Autodesk Fusion 360 part; units mm, degrees
(part 2 of 2)
sketch "Sketch5 (5)" plane through (85, 0, 0) normal (1, 0, 0) x (0, 0, -1) in component "Top"
  line L0 (-100, 190) -> (-100, 195)
  line L1 (-100, 195) -> (-145, 195)
  line L2 (-145, 195) -> (-145, 156)
  line L3 (-145, 156) -> (-150, 156)
  line L4 (-150, 156) -> (-150, 117)
  line L5 (-150, 117) -> (-145, 117)
  line L6 (-145, 117) -> (-145, 78)
  line L7 (-145, 78) -> (-150, 78)
  line L8 (-150, 78) -> (-150, 39)
  line L9 (-150, 39) -> (-145, 39)
  line L10 (-145, 39) -> (-145, 5)
  line L11 (-145, 5) -> (-100, 5)
  line L12 (-100, 5) -> (-100, 0)
  line L13 (-100, 0) -> (-50, 0)
  line L14 (-50, 0) -> (-50, 5)
  line L15 (-50, 5) -> (-5, 5)
  line L16 (-5, 5) -> (-5, 39)
  line L17 (-5, 39) -> (0, 39)
  line L18 (0, 39) -> (0, 78)
  line L19 (0, 78) -> (-5, 78)
  line L20 (-5, 78) -> (-5, 117)
  line L21 (-5, 117) -> (0, 117)
  line L22 (0, 117) -> (0, 156)
  line L23 (0, 156) -> (-5, 156)
  line L24 (-5, 156) -> (-5, 195)
  line L25 (-5, 195) -> (-50, 195)
  line L26 (-50, 195) -> (-50, 190)
  line L27 (-50, 190) -> (-100, 190)
  line L28 (-85, 117) -> (-80, 117)
  line L29 (-80, 117) -> (-80, 78)
  line L30 (-80, 78) -> (-85, 78)
  line L31 (-85, 78) -> (-85, 117)
sketch "Sketch6 (3)" plane through (85, 0, 0) normal (1, 0, 0) x (0, 0, -1) in component "Top"
  line L0 (-100, 190) -> (-100, 195)
  line L1 (-100, 195) -> (-145, 195)
  line L2 (-145, 195) -> (-145, 156)
  line L3 (-145, 156) -> (-150, 156)
  line L4 (-150, 156) -> (-150, 117)
  line L5 (-150, 117) -> (-145, 117)
  line L6 (-145, 117) -> (-145, 78)
  line L7 (-145, 78) -> (-150, 78)
  line L8 (-150, 78) -> (-150, 39)
  line L9 (-150, 39) -> (-145, 39)
  line L10 (-145, 39) -> (-145, 5)
  line L11 (-145, 5) -> (-100, 5)
  line L12 (-100, 5) -> (-100, 0)
  line L13 (-100, 0) -> (-50, 0)
  line L14 (-50, 0) -> (-50, 5)
  line L15 (-50, 5) -> (-5, 5)
  line L16 (-5, 5) -> (-5, 39)
  line L17 (-5, 39) -> (0, 39)
  line L18 (0, 39) -> (0, 78)
  line L19 (0, 78) -> (-5, 78)
  line L20 (-5, 78) -> (-5, 117)
  line L21 (-5, 117) -> (0, 117)
  line L22 (0, 117) -> (0, 156)
  line L23 (0, 156) -> (-5, 156)
  line L24 (-5, 156) -> (-5, 195)
  line L25 (-5, 195) -> (-50, 195)
  line L26 (-50, 195) -> (-50, 190)
  line L27 (-50, 190) -> (-100, 190)
  line L28 (-85, 117) -> (-80, 117)
  line L29 (-80, 117) -> (-80, 78)
  line L30 (-80, 78) -> (-85, 78)
  line L31 (-85, 78) -> (-85, 117)
sketch "Sketch7 (3)" plane through (85, 0, 0) normal (1, 0, 0) x (0, 0, -1) in component "Top"
  line L0 (-100, 190) -> (-100, 195)
  line L1 (-100, 195) -> (-145, 195)
  line L2 (-145, 195) -> (-145, 156)
  line L3 (-145, 156) -> (-150, 156)
  line L4 (-150, 156) -> (-150, 117)
  line L5 (-150, 117) -> (-145, 117)
  line L6 (-145, 117) -> (-145, 78)
  line L7 (-145, 78) -> (-150, 78)
  line L8 (-150, 78) -> (-150, 39)
  line L9 (-150, 39) -> (-145, 39)
  line L10 (-145, 39) -> (-145, 5)
  line L11 (-145, 5) -> (-100, 5)
  line L12 (-100, 5) -> (-100, 0)
  line L13 (-100, 0) -> (-50, 0)
  line L14 (-50, 0) -> (-50, 5)
  line L15 (-50, 5) -> (-5, 5)
  line L16 (-5, 5) -> (-5, 39)
  line L17 (-5, 39) -> (0, 39)
  line L18 (0, 39) -> (0, 78)
  line L19 (0, 78) -> (-5, 78)
  line L20 (-5, 78) -> (-5, 117)
  line L21 (-5, 117) -> (0, 117)
  line L22 (0, 117) -> (0, 156)
  line L23 (0, 156) -> (-5, 156)
  line L24 (-5, 156) -> (-5, 195)
  line L25 (-5, 195) -> (-50, 195)
  line L26 (-50, 195) -> (-50, 190)
  line L27 (-50, 190) -> (-100, 190)
  line L28 (-85, 117) -> (-80, 117)
  line L29 (-80, 117) -> (-80, 78)
  line L30 (-80, 78) -> (-85, 78)
  line L31 (-85, 78) -> (-85, 117)
sketch "Div2" plane through (85, 0, 0) normal (1, 0, 0) x (0, 0, -1)
  line L0 (-100, 190) -> (-100, 195)
  line L1 (-100, 195) -> (-145, 195)
  line L2 (-145, 195) -> (-145, 156)
  line L3 (-145, 156) -> (-150, 156)
  line L4 (-150, 156) -> (-150, 117)
  line L5 (-150, 117) -> (-145, 117)
  line L6 (-145, 117) -> (-145, 78)
  line L7 (-145, 78) -> (-150, 78)
  line L8 (-150, 78) -> (-150, 39)
  line L9 (-150, 39) -> (-145, 39)
  line L10 (-145, 39) -> (-145, 5)
  line L11 (-145, 5) -> (-100, 5)
  line L12 (-100, 5) -> (-100, 0)
  line L13 (-100, 0) -> (-50, 0)
  line L14 (-50, 0) -> (-50, 5)
  line L15 (-50, 5) -> (-5, 5)
  line L16 (-5, 5) -> (-5, 39)
  line L17 (-5, 39) -> (0, 39)
  line L18 (0, 39) -> (0, 78)
  line L19 (0, 78) -> (-5, 78)
  line L20 (-5, 78) -> (-5, 117)
  line L21 (-5, 117) -> (0, 117)
  line L22 (0, 117) -> (0, 156)
  line L23 (0, 156) -> (-5, 156)
  line L24 (-5, 156) -> (-5, 195)
  line L25 (-5, 195) -> (-50, 195)
  line L26 (-50, 195) -> (-50, 190)
  line L27 (-50, 190) -> (-100, 190)
  line L28 (-85, 117) -> (-80, 117)
  line L29 (-80, 117) -> (-80, 78)
  line L30 (-80, 78) -> (-85, 78)
  line L31 (-85, 78) -> (-85, 117)
sketch "Div4" plane through (255, 0, 85) normal (0, 0, 1) x (1, 0, 0)
  line L0 (-250, 5) -> (-237.5, 5)
  line L1 (-237.5, 5) -> (-237.5, 0)
  line L2 (-237.5, 0) -> (-187.5, 0)
  line L3 (-187.5, 0) -> (-187.5, 5)
  line L4 (-187.5, 5) -> (-175, 5)
  line L5 (-175, 5) -> (-175, 78)
  line L6 (-175, 78) -> (-170, 78)
  line L7 (-170, 78) -> (-170, 117)
  line L8 (-170, 117) -> (-175, 117)
  line L9 (-175, 117) -> (-175, 190)
  line L10 (-175, 190) -> (-250, 190)
  line L11 (-250, 190) -> (-250, 117)
  line L12 (-250, 117) -> (-255, 117)
  line L13 (-255, 117) -> (-255, 78)
  line L14 (-255, 78) -> (-250, 78)
  line L15 (-250, 78) -> (-250, 5)
sketch "Bottom" plane through (0, 0, 0) normal (0, -1, 0) x (1, 0, 0)
  line L0 (67.5, 85) -> (67.5, 80)
  line L1 (67.5, 80) -> (17.5, 80)
  line L2 (17.5, 80) -> (17.5, 85)
  line L3 (17.5, 85) -> (67.5, 85)
  line L4 (80, 50) -> (80, 100)
  line L5 (80, 100) -> (85, 100)
  line L6 (85, 100) -> (85, 50)
  line L7 (85, 50) -> (80, 50)
  line L8 (295, 50) -> (295, 100)
  line L9 (295, 100) -> (300, 100)
  line L10 (300, 100) -> (300, 145)
  line L11 (300, 145) -> (250, 145)
  line L12 (250, 145) -> (250, 150)
  line L13 (250, 150) -> (200, 150)
  line L14 (200, 150) -> (200, 145)
  line L15 (200, 145) -> (150, 145)
  line L16 (150, 145) -> (150, 150)
  line L17 (150, 150) -> (100, 150)
  line L18 (100, 150) -> (100, 145)
  line L19 (100, 145) -> (50, 145)
  line L20 (50, 145) -> (50, 150)
  line L21 (50, 150) -> (0, 150)
  line L22 (0, 150) -> (0, 100)
  line L23 (0, 100) -> (5, 100)
  line L24 (5, 100) -> (5, 50)
  line L25 (5, 50) -> (0, 50)
  line L26 (0, 50) -> (0, 0)
  line L27 (0, 0) -> (50, 0)
  line L28 (50, 0) -> (50, 5)
  line L29 (50, 5) -> (100, 5)
  line L30 (100, 5) -> (100, 0)
  line L31 (100, 0) -> (150, 0)
  line L32 (150, 0) -> (150, 5)
  line L33 (150, 5) -> (200, 5)
  line L34 (200, 5) -> (200, 0)
  line L35 (200, 0) -> (250, 0)
  line L36 (250, 0) -> (250, 5)
  line L37 (250, 5) -> (300, 5)
  line L38 (300, 5) -> (300, 50)
  line L39 (300, 50) -> (295, 50)
sketch "Right" plane through (300, 0, 0) normal (1, 0, 0) x (0, 0, -1)
  line L0 (-150, 156) -> (-145, 156)
  line L1 (-145, 156) -> (-145, 117)
  line L2 (-145, 117) -> (-150, 117)
  line L3 (-150, 117) -> (-150, 78)
  line L4 (-150, 78) -> (-145, 78)
  line L5 (-145, 78) -> (-145, 39)
  line L6 (-145, 39) -> (-150, 39)
  line L7 (-150, 39) -> (-150, 0)
  line L8 (-150, 0) -> (-145, 0)
  line L9 (-145, 0) -> (-145, 5)
  line L10 (-145, 5) -> (-100, 5)
  line L11 (-100, 5) -> (-100, 0)
  line L12 (-100, 0) -> (-50, 0)
  line L13 (-50, 0) -> (-50, 5)
  line L14 (-50, 5) -> (-5, 5)
  line L15 (-5, 5) -> (-5, 0)
  line L16 (-5, 0) -> (0, 0)
  line L17 (0, 0) -> (0, 39)
  line L18 (0, 39) -> (-5, 39)
  line L19 (-5, 39) -> (-5, 78)
  line L20 (-5, 78) -> (0, 78)
  line L21 (0, 78) -> (0, 117)
  line L22 (0, 117) -> (-5, 117)
  line L23 (-5, 117) -> (-5, 156)
  line L24 (-5, 156) -> (0, 156)
  line L25 (0, 156) -> (0, 195)
  line L26 (0, 195) -> (-145, 195)
  line L27 (-145, 195) -> (-150, 195)
  line L28 (-150, 195) -> (-150, 156)
  line L29 (-150, 195) -> (-150, 156)
  line L30 (0, 156) -> (0, 195)
  line L31 (-100, 0) -> (-50, 0)
  line L32 (-150, 156) -> (-150, 117)
  dimension "d152" = 150
  dimension "d153" = 195
  dimension "d154" = 39
  measures "d152" distance of L29 L30
  measures "d153" distance of L26 L31
  measures "d154" distance of L0.start L2.end
component "Right" placed x (1, 0, 0) y (0, 1, 0) z (0, 0, 1) at (0, 0, 0)
component "Left" placed x (1, 0, 0) y (0, 1, 0) z (0, 0, 1) at (0, 0, 0)
component "Back" placed x (1, 0, 0) y (0, 1, 0) z (0, 0, 1) at (0, 0, 0)
component "Front" placed x (1, 0, 0) y (0, 1, 0) z (0, 0, 1) at (0, 0, 0)
component "Divider2" placed x (1, 0, 0) y (0, 1, 0) z (0, 0, 1) at (0, 0, 0)
component "Base" placed x (1, 0, 0) y (0, 1, 0) z (0, 0, 1) at (0, 0, 0)
component "Divider4" placed x (1, 0, 0) y (0, 1, 0) z (0, 0, 1) at (0, 0, 75)
component "Top" placed x (1, 0, 0) y (0, 1, 0) z (0, 0, 1) at (0, 0, 0)
equation "t = 5 mm"
equation "d27 = -t"
equation "d43 = -t"
equation "d65 = -t"
equation "d69 = -t"
equation "d84 = -t"
equation "d93 = -t"
equation "d107 = -t"
equation "d114 = -t"
equation "d116 = -t"
equation "d122 = -t"
equation "d124 = -t"
equation "d129 = -t"
equation "d131 = t"
equation "d134 = t"
equation "d136 = t"
equation "d138 = t"
equation "d140 = -t"
equation "d141 = -t"
equation "d143 = -t"
equation "d148 = -t"
equation "d150 = t"
